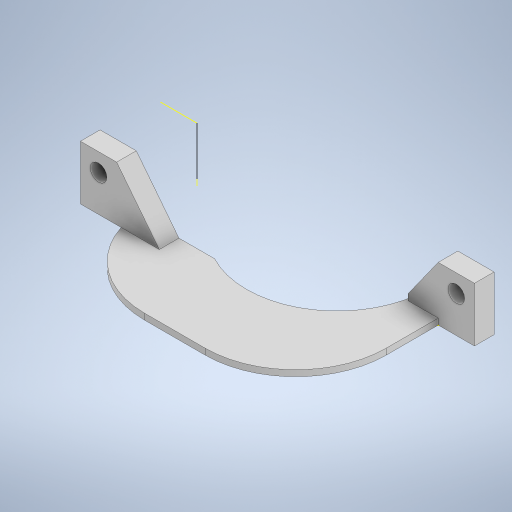
# Autodesk Inventor part: PartsForRaspibase
Saved by Autodesk Inventor 2024.2 (Build 282272000, 272)
## iProperties
Created: 2024-04-03
Part Number: PartsForRaspibase
Material: 一般
Document SubType Name: Modeling
Designer: yukin
Density: 1 g/cm^3
Appearance: 既定
Author: yukin
Autodesk Inventor part; units mm, degrees
ref_plane "YZ Plane" through (0, 0, 0) normal (1, 0, 0) x (0, 1, 0)
ref_plane "XZ Plane" through (0, 0, 0) normal (0, 1, 0) x (-1, 0, 0)
ref_plane "XY Plane" through (0, 0, 0) normal (0, 0, 1) x (1, 0, 0)
sketch "スケッチ1" plane through (0, 0, 0) normal (0, 1, 0) x (-1, 0, 0)
  line L0 (0, 0) -> (40, 0)
  line L1 (40, 0) -> (40, -26.8558)
  line L2 (40, -26.8558) -> (0, -26.8558)
  line L3 (0, -26.8558) -> (0, 0)
  circle A0 centre (20, -26.8558) radius 15
  line L4 (20, -26.8558) -> (20, 0)
  line L5 (40, -23.6058) -> (40, -26.8558)
  line L6 (0, -23.6058) -> (0, -26.8558)
  circle A1 centre (20, -26.8558) radius 17
  line L7 (40, -26.8558) -> (46, -26.8558)
  line L8 (46, -26.8558) -> (46, -23.6058)
  line L9 (46, -23.6058) -> (40, -23.6058)
  line L10 (40, -23.6058) -> (40, -26.8558)
  line L11 (0, -23.6058) -> (0, -26.8558)
  line L12 (0, -26.8558) -> (-6, -26.8558)
  line L13 (-6, -26.8558) -> (-6, -23.6058)
  line L14 (-6, -23.6058) -> (0, -23.6058)
  line L15 (0, -23.6058) -> (0, -26.8558)
  point P0 (35, -26.8558)
  point P1 (5, -26.8558)
  dimension "d0" = 40
  dimension "d1" = 30
  dimension "d16" = 34
  dimension "d18" = 6
  dimension "d19" = 3.25
  constraints: 32 end point, 5 symmetric about line, 4 parallel, 2 centre point, 2 horizontal, 2 midpoint, 2 perpendicular, 1 coincident
  measures "d0" distance of L1.end L2.end
  measures "d1" diameter of A0
  measures "d16" diameter of A1
  measures "d18" distance of L9.end L8.end
  measures "d19" distance of L8.end L7.end
extrude "押し出し1" add sketch "スケッチ1" along normal blind 1 contours L0 L4 A1 L2 L3 | L0 L1 L2 A1 L4 | A1 L2 A0 L4 | L4 A0 L2 A1 | L4 L2 A0 | A0 L2 L4
fillet "フィレット1" radius 15 2 edges at (-40, 0.5, 0) (0, 0.5, 0)
extrude "押し出し4" add sketch "スケッチ1" along normal blind 9 contours L3 L12 L13 L14 | L9 L8 L7 L1
sketch "スケッチ7" plane through (6, 0, -26.8558) normal (0, 0, -1) x (-1, 0, 0)
  circle A0 centre (3, 6) radius 1.375
  line L0 (6, 1) -> (6, 9) projected
  line L1 (0, 9) -> (6, 9) projected
  circle A1 centre (49.4019, 6) radius 1.375
  line L2 (46, 9) -> (52, 9) projected
  line L3 (52, 0) -> (52, 9) projected
  point P0 (6, 0)
  point P1 (3, 9)
  point P2 (52, 4.5)
  dimension "d22" = 2.75
  dimension "d23" = 3
  dimension "d24" = 3
  dimension "d25" = 2.75
  dimension "d26" = 3
  dimension "d27" = 3
  constraints: 2 centre point, 2 midpoint
  measures "d22" diameter of A0
  measures "d23" distance from line of L0 A0.centre
  measures "d24" distance of A0.centre point (3, 9)
  measures "d25" diameter of A1
  measures "d26" distance from line of A1.centre L2
  measures "d27" distance of point (52, 4.5) A1.centre
extrude "押し出し5" cut sketch "スケッチ7" against normal blind 6
extrude "押し出し6" cut sketch "スケッチ1" along normal blind 1 contours L4 L2 A0 | A0 L2 L4
sketch "スケッチ9" plane through (6, 9, -26.8558) normal (0, 0, -1) x (-1, 0, 0)
  line L0 (6, -8) -> (6, 0) projected
  line L1 (6, -8) -> (11, -8)
  line L2 (11, -8) -> (11, -7)
  line L3 (11, -7) -> (6, -7)
  line L4 (6, -7) -> (6, -8)
  line L5 (6, 0) -> (11, -7)
  line L6 (41, -8) -> (41, -9) projected
  line L7 (52, 0) -> (46, 0) projected
  line L8 (46, -8) -> (46, 0) projected
  line L9 (46, -8) -> (41, -8)
  line L10 (41, -8) -> (41, -7)
  line L11 (41, -7) -> (46, -7)
  line L12 (46, -7) -> (46, -8)
  line L13 (46, 0) -> (41, -7)
  point P0 (6, -9)
  dimension "d32" = 5
  dimension "d33" = 1
  dimension "d38" = 5
  constraints: 20 end point, 4 parallel, 2 horizontal, 2 perpendicular
  measures "d32" distance of L3.end L2.end
  measures "d33" distance of L2.end L1.end
  measures "d38" distance of L10.end L11.end
extrude "押し出し7" add sketch "スケッチ9" against normal blind 3.25
sketch "スケッチ10" plane through (0, 1, 0) normal (0, 1, 0) x (1, 0, 0)
  line L0 (-35, 23.6058) -> (-40, 23.6058) projected
  line L1 (-40, 23.6058) -> (-35, 23.6058)
  line L2 (-35, 23.6058) -> (-35, 13.6058)
  line L3 (-35, 13.6058) -> (-40, 13.6058)
  line L4 (-40, 13.6058) -> (-40, 23.6058)
  line L5 (-40, 13.6058) -> (-27, 13.6058)
  line L6 (-27, 13.6058) -> (-27, 10.3558)
  line L7 (-27, 10.3558) -> (-40, 10.3558)
  line L8 (-40, 10.3558) -> (-40, 13.6058)
  line L9 (-24.5918, 17.2551) -> (-23.5955, 17.2551)
  line L10 (-23.5955, 17.2551) -> (-23.5955, 14.4656)
  line L11 (-23.5955, 14.4656) -> (-24.5918, 14.4656)
  line L12 (-24.5918, 14.4656) -> (-24.5918, 17.2551)
  arc A0 (-40, 15) -> (-25, 0) centre (-25, 15) ccw projected
  arc A1 (-40, 15) -> (-39.2629, 10.3558) centre (-25, 15) ccw
  line L13 (-40, 13.6058) -> (-46, 13.6058)
  line L14 (-46, 13.6058) -> (-46, 10.3558)
  line L15 (-46, 10.3558) -> (-40, 10.3558)
  line L16 (-40, 10.3558) -> (-40, 13.6058)
  point P0 (0, 0)
  dimension "d39" = 5
  dimension "d40" = 10
  dimension "d41" = 13
  dimension "d42" = 3.25
  dimension "d43" = 6
  constraints: 32 end point, 8 parallel, 4 horizontal, 4 perpendicular, 3 point on circle, 1 centre point, 1 point on line
  measures "d39" distance of L2.end L3.end
  measures "d40" distance of L1.end L2.end
  measures "d41" distance of L6.end L7.end
  measures "d42" distance of L5.end L6.end
  measures "d43" distance of L15.end L14.end
sketch "スケッチ11" plane through (-46, 0, -23.6058) normal (0, 0, 1) x (1, 0, 0)
  line L0 (0, 9) -> (6, 9) projected
  line L1 (6, 1) -> (6, 0) projected
  line L2 (6, 9) -> (6, 1)
  point P0 (46, 0)
  constraints: 2 end point, 1 collinear
extrude "押し出し8" add sketch "スケッチ10" along normal blind 9 contours L8 L15 L14 L13
sketch "スケッチ12" plane through (-46, 1, -10.3558) normal (0, 0, 1) x (1, 0, 0)
  line L0 (0, 0) -> (6, 0) projected
  line L1 (6, 0) -> (13.0551, 0)
  line L2 (0, 9) -> (6, 9) projected
  line L3 (13.0551, 0) -> (6, 9)
  line L4 (6, 0) -> (6, 9) projected
  line L5 (6, 0) -> (6, 9)
  point P0 (46, -1)
  constraints: 6 end point, 1 horizontal, 1 vertical
extrude "押し出し9" add sketch "スケッチ12" against normal blind 3.25
sketch "スケッチ13" plane through (-46, 1, -10.3558) normal (0, 0, 1) x (1, 0, 0)
  circle A0 centre (3, 6) radius 1.375
  line L0 (0, 9) -> (6, 9) projected
  line L1 (0, 0) -> (0, 9) projected
  point P0 (46, -1)
  dimension "d48" = 2.75
  dimension "d49" = 3
  dimension "d50" = 3
  constraints: 1 centre point
  measures "d48" diameter of A0
  measures "d49" distance from line of L0 A0.centre
  measures "d50" distance from line of L1 A0.centre
extrude "押し出し10" cut sketch "スケッチ13" against normal blind 3.25
sketch "スケッチ14" plane through (-46, 0, -23.6058) normal (0, 0, 1) x (1, 0, 0)
  line L0 (11, 1) -> (11, 2) projected
  line L1 (0, 9) -> (6, 9) projected
  line L2 (11, 1) -> (0, 1)
  line L3 (0, 1) -> (0, 9)
  line L4 (0, 9) -> (11, 9)
  line L5 (11, 9) -> (11, 1)
  line L6 (0, 1) -> (6, 1)
  line L7 (6, 1) -> (6, 0)
  line L8 (6, 0) -> (0, 0)
  line L9 (0, 0) -> (0, 1)
  point P0 (46, 0)
  constraints: 16 end point, 4 parallel, 2 horizontal, 2 perpendicular
extrude "押し出し11" cut sketch "スケッチ14" against normal blind 9
sketch "スケッチ15" plane through (0, 1, 0) normal (0, 1, 0) x (1, 0, 0)
  arc A0 (-40, 15) -> (-39.9351, 13.6058) centre (-25, 15) ccw projected
  line L0 (-39.9351, 13.6058) -> (-27.0312, 13.6058)
  arc A1 (-35, 26.8558) -> (-5, 26.8558) centre (-20, 26.8558) ccw projected
  line L1 (-39.9351, 13.6058) -> (-32.9449, 13.6058) projected
  line L2 (-40, 26.8558) -> (-40, 15) projected
  line L3 (-39.9351, 13.6058) -> (-40, 26.8558)
  line L4 (-40, 26.8558) -> (-35, 26.8558) projected
  line L5 (-40, 26.8558) -> (-35, 26.8558)
  line L6 (-35, 26.8558) -> (-27.0312, 13.6058)
  arc A2 (-39.9351, 13.6058) -> (-39.2629, 10.3558) centre (-25, 15) ccw projected
  arc A3 (-40, 26.8558) -> (-39.9351, 13.6058) centre (466.0679, 22.7107) ccw
  point P0 (0, 0)
  point P1 (-40, 18.5657)
  constraints: 8 end point, 3 point on circle, 1 centre point, 1 collinear, 1 horizontal
extrude "押し出し12" cut sketch "スケッチ15" against normal blind 9 contours L3 L4 A1 L0 | A3 L2 L3
sketch "スケッチ16" plane through (0, 1, 0) normal (0, 1, 0) x (1, 0, 0)
  arc A0 (-40, 15) -> (-39.9351, 13.6058) centre (-25, 15) ccw projected
  line L0 (-40, 18.5657) -> (-40, 15) projected
  line L1 (-39.9351, 13.6058) -> (-40, 18.5657)
  arc A1 (-40, 18.5657) -> (-39.9351, 13.6058) centre (0.7021, 16.6182) ccw
  point P0 (0, 0)
  constraints: 2 end point, 2 point on circle, 1 centre point
extrude "押し出し13" cut sketch "スケッチ16" against normal blind 9 contours L0 L1 A1 A0 | A0 A1 L0
sketch "スケッチ17" plane through (0, 1, 0) normal (0, 1, 0) x (1, 0, 0)
  arc A0 (-39.992, 14.51) -> (-39.9351, 13.6058) centre (-25, 15) ccw projected
  line L0 (-39.9351, 13.6058) -> (-27.0312, 13.6058) projected
  line L1 (-39.992, 14.51) -> (-39.9351, 14.51)
  line L2 (-39.9351, 14.51) -> (-39.9351, 13.6058)
  line L3 (-39.9351, 13.6058) -> (-39.992, 13.6058)
  line L4 (-39.992, 13.6058) -> (-39.992, 14.51)
  point P0 (0, 0)
  constraints: 8 end point, 2 parallel, 1 horizontal, 1 perpendicular
extrude "押し出し14" cut sketch "スケッチ17" against normal blind 9
